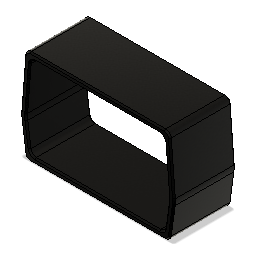
Pojistka autopásu v4 (Autodesk Fusion 360 design; units mm, degrees)
Autodesk Fusion 360 part; units mm, degrees
sketch "Sketch1" plane through (0, 0, 0) normal (0, 0, 1) x (1, 0, 0)
  line L0 (0, 25) -> (0, -25)
  line L1 (0, 21.0169) -> (-24, 21.0169)
  line L2 (-24, 21.0169) -> (-25.5, 2.0169)
  line L3 (-25.5, 2.0169) -> (-24, -8.9831)
  line L4 (-24, -8.9831) -> (0, -8.9831)
  line L5 (0, 23.0169) -> (-25.8483, 23.0169)
  line L6 (-25.8483, 23.0169) -> (-27.5107, 1.9598)
  line L7 (-27.5107, 1.9598) -> (-25.7458, -10.9831)
  line L8 (-25.7458, -10.9831) -> (0, -10.9831)
  line L9 (-25.5, 2.0169) -> (0, 2.0169)
  line L10 (0, 13.5169) -> (-5, 13.5169)
  line L11 (-5, 13.5169) -> (-5, 9.5169)
  line L12 (-5, 9.5169) -> (0, 9.5169)
  line L13 (0, 21.0169) -> (0, 2.0169) construction
  line L14 (27.5107, 1.9598) -> (25.7458, -10.9831)
  line L15 (25.7458, -10.9831) -> (0, -10.9831)
  line L16 (25.8483, 23.0169) -> (27.5107, 1.9598)
  line L17 (0, 21.0169) -> (24, 21.0169)
  line L18 (25.5, 2.0169) -> (24, -8.9831)
  line L19 (24, -8.9831) -> (0, -8.9831)
  line L20 (24, 21.0169) -> (25.5, 2.0169)
  line L21 (0, 23.0169) -> (25.8483, 23.0169)
  line L22 (5, 13.5169) -> (5, 9.5169)
  line L23 (5, 9.5169) -> (0, 9.5169)
  line L24 (0, 13.5169) -> (5, 13.5169)
  line L25 (25.5, 2.0169) -> (0, 2.0169)
  point P0 (-5, 11.5169)
  point P1 (0, 11.5169)
  dimension "d1" = 51
  dimension "d2" = 48
  dimension "d3" = 48
  dimension "d4" = 30
  dimension "d5" = 19
  dimension "d7" = 2
  dimension "d8" = 19
  dimension "d9" = 4
  dimension "d11" = 10
  constraint vertical L0
  constraint coincident L0 L1.start
  constraint perpendicular L0 L1
  constraint coincident L0 L4.end
  constraint perpendicular L0 L4
  constraint coincident L0 L9.end
  constraint perpendicular L0 L9
  constraint coincident L2 L3.start
  constraint coincident L0 L10.start
  constraint perpendicular L0 L10
  constraint perpendicular L10 L11
  constraint coincident L0 L12.end
  constraint perpendicular L11 L12
  constraint midpoint L11 P0
  constraint midpoint L13 P1
  constraint horizontal P0 P1
  constraint symmetric L0 L1.start L13.start
  constraint symmetric L0 L1.end L17.end
  constraint symmetric L0 L2.end L18.start
  constraint symmetric L0 L3.end L18.end
  constraint symmetric L0 L4.end L19.end
  constraint symmetric L0 L5.start L21.start
  constraint symmetric L0 L5.end L16.start
  constraint symmetric L0 L6.end L14.start
  constraint symmetric L0 L7.end L14.end
  constraint symmetric L0 L8.end L15.end
  constraint symmetric L0 L10.start L24.start
  constraint symmetric L0 L10.end L22.start
  constraint symmetric L0 L11.end L22.end
  constraint symmetric L0 L12.end L23.end
  constraint symmetric L0 L9.end L13.end
  measures "d4" distance of L1 L4
  measures "d5" distance of L1 L2.end
  measures "d8" distance of L1 L9
  measures "d9" distance of L10.end L11.end
extrude "Extrude1" add sketch "Sketch1" against normal blind 2 contours L0 L14 L15 L16 L17 L18 L19 L20 L21 | L0 L1 L2 L3 L4 L5 L6 L7 L8 | L0 L17 L20 L22 L23 L24 L25 | L0 L1 L2 L9 L10 L11 L12
extrude "Extrude2" add sketch "Sketch1" along normal blind 20 contours L0 L14 L15 L16 L17 L18 L19 L20 L21 | L0 L1 L2 L3 L4 L5 L6 L7 L8
fillet "Fillet1" radius 2 8 edges at (-25.8483, 23.0169, 9) (25.8483, 23.0169, 9) (25.7458, -10.9831, 9) (-25.7458, -10.9831, 9) (-24, 21.0169, 10) (24, 21.0169, 10) (24, -8.9831, 9) (-24, -8.9831, 9)
fillet "Fillet1" radius 10 4 edges at (25.5, 2.0169, 10) (-25.5, 2.0169, 10) (27.5107, 1.9598, 9) (-27.5107, 1.9598, 9)
chamfer "Chamfer1" distance 0.5 angle 45 1 faces at (18.812, 12.236, -2)
chamfer "Chamfer1" distance 0.5 angle 45 1 faces at (18.1869, 10.5934, 0)
chamfer "Chamfer1" distance 0.5 angle 45 1 faces at (-7.3839, 22.3502, 20)
equation "t = 2 mm" comment "Síla stěny"
equation "d7 = t"
equation "d12 = -t"
equation "d17 = t"
named bodies: "Pojistka"
